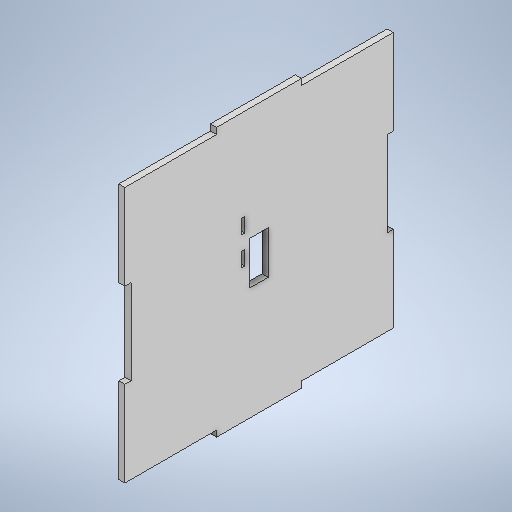
# Autodesk Inventor part: TOPO DO POÇO 6 mm (fixed)
Saved by Autodesk Inventor 2025.2 (Build 292293000, 293)
## iProperties
Created: 2025-05-08
Part Number: TOPO DO POÇO 6 mm (fixed)
Material: Genérico
Document SubType Name: Modeling
Designer: erick
Density: 1 g/cm^3
Appearance: Padrão
Author: erick
Autodesk Inventor part; units mm, degrees
ref_plane "YZ Plane" through (0, 0, 0) normal (1, 0, 0) x (0, 1, 0)
ref_plane "XZ Plane" through (0, 0, 0) normal (0, 1, 0) x (-1, 0, 0)
ref_plane "XY Plane" through (0, 0, 0) normal (0, 0, 1) x (1, 0, 0)
sketch "Esboço1" plane through (0, 0, 0) normal (1, 0, 0) x (0, 1, 0)
  line L0 (-131, 131) -> (131, 131)
  line L1 (131, 131) -> (131, -131)
  line L2 (131, -131) -> (-131, -131)
  line L3 (-131, -131) -> (-131, 131)
  line L4 (-131, 131) -> (131, -131) construction
  line L5 (131, 131) -> (-131, -131) construction
  line L6 (-15, 9) -> (15, 9)
  line L7 (15, 9) -> (15, -9)
  line L8 (15, -9) -> (-15, -9)
  line L9 (-15, -9) -> (-15, 9)
  line L10 (-15, 9) -> (15, -9) construction
  line L11 (15, 9) -> (-15, -9) construction
  point P0 (0, 0)
  dimension "d0" = 262
  dimension "d1" = 262
  dimension "d35" = 30
  dimension "d36" = 18
  constraints: 24 end point, 4 midpoint, 4 parallel, 2 horizontal, 2 perpendicular
  measures "d0" distance of L0.end L1.end
  measures "d1" distance of L1.end L2.end
  measures "d35" distance of L7.end L8.end
  measures "d36" distance of L6.end L7.end
extrude "Extrusão1" add sketch "Esboço1" along normal mid plane 6 contours L0 L1 L2 L3 | L6 L7 L8 L9
sketch "Esboço2" plane through (3, 0, 0) normal (1, 0, 0) x (0, 0, -1)
  line L0 (131, 131) -> (-131, 131) projected
  line L1 (-131, 131) -> (-41.5, 131)
  line L2 (-41.5, 131) -> (-41.5, 125)
  line L3 (-41.5, 125) -> (-131, 125)
  line L4 (-131, 125) -> (-131, 131)
  line L5 (131, 131) -> (41.5, 131)
  line L6 (41.5, 131) -> (41.5, 125)
  line L7 (41.5, 125) -> (131, 125)
  line L8 (131, 125) -> (131, 131)
  line L9 (-131, 131) -> (-131, -131) projected
  line L10 (-131, -131) -> (-41.5, -131)
  line L11 (-41.5, -131) -> (-41.5, -125)
  line L12 (-41.5, -125) -> (-131, -125)
  line L13 (-131, -125) -> (-131, -131)
  line L14 (131, -131) -> (131, 131) projected
  line L15 (131, -131) -> (41.5, -131)
  line L16 (41.5, -131) -> (41.5, -125)
  line L17 (41.5, -125) -> (131, -125)
  line L18 (131, -125) -> (131, -131)
  point P0 (0, 0)
  point P1 (131, -125)
  point P2 (-131, -125)
  point P3 (41.5, 131)
  dimension "d4" = 89.5
  dimension "d5" = 6
  dimension "d6" = 89.5
  dimension "d7" = 6
  dimension "d8" = 83
  dimension "d9" = 89.5
  dimension "d10" = 6
  dimension "d11" = 89.5
  dimension "d12" = 6
  dimension "d13" = 83
  constraints: 32 end point, 8 parallel, 4 horizontal, 4 perpendicular
  measures "d4" distance of L2.end L3.end
  measures "d5" distance of L1.end L2.end
  measures "d6" distance of L6.end L7.end
  measures "d7" distance of L5.end L6.end
  measures "d8" distance between parallel lines of L6 L2
  measures "d9" distance of L11.end L12.end
  measures "d10" distance of L10.end L11.end
  measures "d11" distance of L16.end L17.end
  measures "d12" distance of L15.end L16.end
  measures "d13" distance between parallel lines of L16 L11
extrude "Extrusão2" cut sketch "Esboço2" along normal through all both and the other way through all
sketch "Esboço3" plane through (3, 0, 0) normal (1, 0, 0) x (0, 0, -1)
  line L0 (-125, 41.5) -> (-137, 41.5)
  line L1 (-137, 41.5) -> (-137, -41.5)
  line L2 (-137, -41.5) -> (-125, -41.5)
  line L3 (-125, -41.5) -> (-125, 41.5)
  line L4 (-131, -125) -> (-131, 125) projected
  line L5 (-125, 41.5) -> (-137, -41.5) construction
  line L6 (-137, 41.5) -> (-125, -41.5) construction
  line L7 (125, -41.5) -> (137, -41.5)
  line L8 (137, -41.5) -> (137, 41.5)
  line L9 (137, 41.5) -> (125, 41.5)
  line L10 (125, 41.5) -> (125, -41.5)
  line L11 (131, 125) -> (131, -125) projected
  line L12 (125, -41.5) -> (137, 41.5) construction
  line L13 (137, -41.5) -> (125, 41.5) construction
  line L14 (-41.5, 125) -> (-131, 125) projected
  line L15 (-131, -125) -> (-41.5, -125) projected
  line L16 (131, 125) -> (41.5, 125) projected
  line L17 (41.5, -125) -> (131, -125) projected
  point P0 (0, 0)
  point P1 (-131, 0)
  point P2 (131, 0)
  dimension "d16" = 83
  dimension "d17" = 12
  dimension "d18" = 12
  dimension "d19" = 83
  dimension "d20" = 83.5
  dimension "d21" = 83.5
  dimension "d22" = 83.5
  dimension "d23" = 83.5
  constraints: 24 end point, 6 midpoint, 4 parallel, 2 horizontal, 2 perpendicular
  measures "d16" distance of L7.end L8.end
  measures "d17" distance of L8.end L9.end
  measures "d18" distance of L0.start L0.end
  measures "d19" distance of L2.end L0.start
  measures "d20" distance between parallel lines of L0 L14
  measures "d21" distance between parallel lines of L15 L2
  measures "d22" distance between parallel lines of L9 L16
  measures "d23" distance between parallel lines of L17 L7
extrude "Extrusão3" cut sketch "Esboço3" along normal through all both and the other way through all
sketch "Esboço7" plane through (3, 0, 0) normal (1, 0, 0) x (0, 0, -1)
  line L0 (-9, 21) -> (9, 21)
  line L1 (9, 21) -> (9, -21)
  line L2 (9, -21) -> (-9, -21)
  line L3 (-9, -21) -> (-9, 21)
  line L4 (-9, 21) -> (9, -21) construction
  line L5 (9, 21) -> (-9, -21) construction
  point P0 (0, 0)
  dimension "d37" = 18
  dimension "d38" = 42
  constraints: 12 end point, 2 midpoint, 2 parallel, 1 horizontal, 1 perpendicular
  measures "d37" distance of L1.end L2.end
  measures "d38" distance of L0.end L1.end
extrude "Extrusão6" cut sketch "Esboço7" against normal through all
sketch "Esboço11" plane through (3, 0, 0) normal (1, 0, 0) x (0, 0, -1)
  line L0 (-17, 0) -> (-14, 0)
  line L1 (-14, 0) -> (-14, 14)
  line L2 (-14, 14) -> (-17, 14)
  line L3 (-17, 14) -> (-17, 0)
  line L4 (-9, -21) -> (-9, 21) projected
  line L5 (-17, 28) -> (-14, 28)
  line L6 (-14, 28) -> (-14, 42)
  line L7 (-14, 42) -> (-17, 42)
  line L8 (-17, 42) -> (-17, 28)
  point P0 (0, 0)
  dimension "d41" = 3
  dimension "d42" = 8
  dimension "d43" = 14
  dimension "d44" = 14
  dimension "d45" = 3
  dimension "d46" = 8
  dimension "d47" = 14
  dimension "d48" = 14
  constraints: 16 end point, 4 parallel, 2 horizontal, 2 perpendicular
  measures "d41" distance of L0.start L0.end
  measures "d42" distance between parallel lines of L4 L3
  measures "d43" distance of L2.end L0.start
  measures "d44" distance of L5.end L6.end
  measures "d45" distance of L6.end L7.end
  measures "d46" distance between parallel lines of L8 L4
  measures "d47" distance between parallel lines of L5 L2
  measures "d48" distance from line of point (0, 0) L2
extrude "Extrusão7" cut sketch "Esboço11" against normal through all
